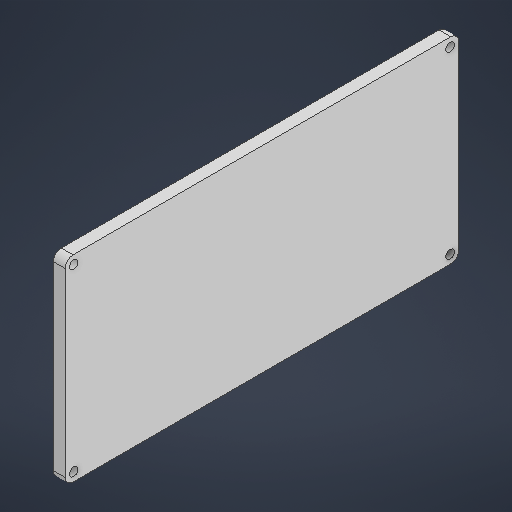
# Autodesk Inventor part: ściana tylna
Saved by Autodesk Inventor 2026.1 (Build 301233020, 233B)
## iProperties
Created: 2026-03-28
Part Number: ściana tylna
Material: Generic
Document SubType Name: Modeling
Designer: Jan
Density: 1 g/cm^3
Appearance: Default
Author: Jan
Autodesk Inventor part; units mm, degrees
ref_plane "YZ Plane" through (0, 0, 0) normal (1, 0, 0) x (0, 1, 0)
ref_plane "XZ Plane" through (0, 0, 0) normal (0, 1, 0) x (-1, 0, 0)
ref_plane "XY Plane" through (0, 0, 0) normal (0, 0, 1) x (1, 0, 0)
sketch "Sketch1" plane through (0, 0, 0) normal (1, 0, 0) x (0, 1, 0)
  line L0 (2, 0) -> (48, 0)
  line L1 (50, -2) -> (50, -98)
  line L2 (48, -100) -> (2, -100)
  line L3 (0, -98) -> (0, -2)
  arc A0 (50, -2) -> (48, 0) centre (48, -2) ccw
  arc A1 (0, -98) -> (2, -100) centre (2, -98) ccw
  arc A2 (48, -100) -> (50, -98) centre (48, -98) ccw
  arc A3 (2, 0) -> (0, -2) centre (2, -2) ccw
  circle A4 centre (47.8, -2.2) radius 1.1
  line L4 (50, -50) -> (19.7358, -50) construction
  line L5 (25, 0) -> (25, -33.4431) construction
  circle A5 centre (47.8, -97.8) radius 1.1
  circle A6 centre (2.2, -2.2) radius 1.1
  circle A7 centre (2.2, -97.8) radius 1.1
  point P0 (0, 0)
  point P1 (50, -100)
  point P2 (50, 0)
  point P3 (0, -100)
  point P4 (2, -2)
  point P5 (2, -98)
  dimension "d0" = 50
  dimension "d1" = 100
  dimension "d2" = 2
  dimension "d3" = 2.2
  dimension "d4" = 2.2
  dimension "d5" = 2.2
  constraints: 12 end point, 8 centre point, 8 point on circle, 8 point on line, 8 tangent, 5 symmetric about line, 3 equal radius, 2 horizontal, 2 midpoint, 2 parallel, 1 perpendicular, 1 vertical, 3 other
  measures "d0" distance of point (50, -100) point (0, -100)
  measures "d1" distance of point (50, 0) point (50, -100)
  measures "d2" radius of A0
  measures "d3" diameter of A4
  measures "d4" distance from line of L1 A4.centre
  measures "d5" distance from line of A4.centre L0
extrude "Extrusion1" add sketch "Sketch1" along normal blind 3 contours L0 A0 L1 A2 L2 A1 L3 A3 | A4 | A5 | A6 | A7
hole "Hole1" at (0, 47.8, -2.2) at (0, 2.2, -2.2) at (0, 47.8, -97.8) at (0, 2.2, -97.8) direction (1, 0, 0) diameter 2.2 depth 6.3 tip angle 118 clearance for "Countersunk Flat Head Screw ISO 2009/7046" size "M2" standard "ISO"
body "Solid1"
